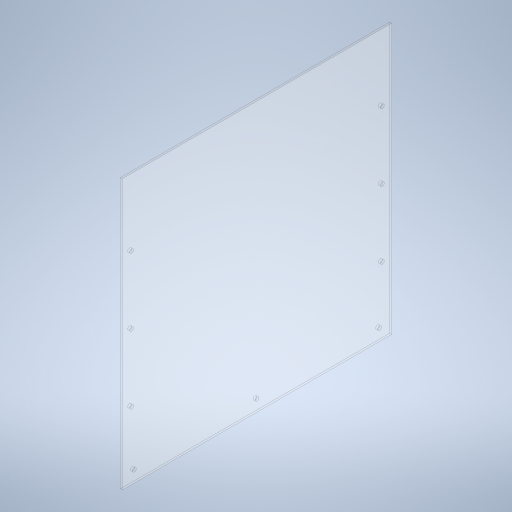
# Autodesk Inventor part: HCMUTE-CDT23-KXL_A02
Saved by Autodesk Inventor 2023 (Build 270158000, 158)
## iProperties
Created: 2023-11-20
Part Number: HCMUTE-CDT23-KXL_A02
Material: PMMA Plastic
Document SubType Name: Modeling
Designer: havie
Density: 1.188 g/cm^3
Appearance: Clear - Light
Author: havie
Autodesk Inventor part; units mm, degrees
ref_plane "YZ Plane" through (0, 0, 0) normal (1, 0, 0) x (0, 1, 0)
ref_plane "XZ Plane" through (0, 0, 0) normal (0, 1, 0) x (-1, 0, 0)
ref_plane "XY Plane" through (0, 0, 0) normal (0, 0, 1) x (1, 0, 0)
sketch "Sketch1" plane through (0, 0, 0) normal (0, 1, 0) x (-1, 0, 0)
  line L0 (-200, 200) -> (200, 200)
  line L1 (200, 200) -> (200, -200)
  line L2 (200, -200) -> (-200, -200)
  line L3 (-200, -200) -> (-200, 200)
  line L4 (-200, 200) -> (200, -200) construction
  line L5 (200, 200) -> (-200, -200) construction
  point P0 (0, 0)
  dimension "d0" = 400
  constraints: 12 end point, 2 midpoint, 2 parallel, 2 perpendicular, 1 horizontal
  measures "d0" distance of L0.end L1.end
extrude "Extrusion1" add sketch "Sketch1" along normal mid plane 3
sketch "Sketch2" plane through (0, -1.5, 0) normal (0, -1, 0) x (1, 0, 0)
  line L0 (-200, -200) -> (200, -200) projected
  point P0 (0, 0)
  point P1 (-182, -183)
  point P2 (0, -183)
  point P3 (182, -183)
  dimension "d3" = 182
  dimension "d4" = 182
  dimension "d5" = 17
  constraints: 2 horizontal alignment, 1 vertical alignment
  measures "d3" distance of point (0, -183) point (-182, -183)
  measures "d4" distance of point (182, -183) point (0, -183)
  measures "d5" distance from line of L0 point (-182, -183)
hole "Hole1" at (-182, -1.5, -183) at (0, -1.5, -183) at (182, -1.5, -183) direction (0, 1, 0) diameter 6 depth 14.2 tip angle 118
sketch "Sketch3" plane through (0, -1.5, 0) normal (0, -1, 0) x (1, 0, 0)
  line L0 (200, 200) -> (-200, 200) projected
  line L1 (-200, 200) -> (-200, -200) projected
  point P0 (0, 0)
  point P1 (-186, 100)
  point P2 (-186, 0)
  point P3 (-186, -100)
  dimension "d13" = 100
  dimension "d14" = 100
  dimension "d15" = 100
  dimension "d16" = 14
  constraints: 2 vertical alignment
  measures "d13" distance from line of L0 point (-186, 100)
  measures "d14" distance of point (-186, 0) point (-186, 100)
  measures "d15" distance of point (-186, -100) point (-186, 0)
  measures "d16" distance from line of point (-186, 100) L1
hole "Hole2" at (-186, -1.5, 100) at (-186, -1.5, 0) at (-186, -1.5, -100) direction (0, 1, 0) diameter 6 depth 14.2 tip angle 118
mirror "Mirror1" about plane through (0, 0, 0) normal (1, 0, 0) of "Hole2"
equation "\"d4\" = d3"
equation "\"d14\" = d13"
equation "\"d15\" = d14"
body "Solid1"
